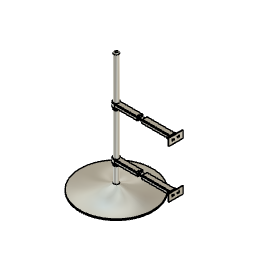
Base & Stand & Arms (Current) v10 (Autodesk Fusion 360 design; units mm, degrees)
Autodesk Fusion 360 part; units mm, degrees
sketch "Sketch1" plane through (0, 0, 0) normal (0, 1, 0) x (1, 0, 0) in component "Base"
  line L0 (0, 0) -> (0, -5)
  line L1 (0, -5) -> (5, -5)
  line L2 (5, -5) -> (5, -15)
  line L3 (5, -15) -> (10, -15)
  line L4 (10, -15) -> (10, -30)
  line L5 (0, 0) -> (150, 0)
  line L6 (150, 0) -> (150, -5)
  arc A0 (150, -5) -> (10, -30) centre (184.7311, -603.994) ccw
  dimension "d1" = 150
  dimension "d2" = 5
  dimension "d3" = 5
  dimension "d4" = 10
  dimension "d5" = 10
  dimension "d6" = 30
  dimension "d7" = 600
  dimension "d8" = 5
  constraint coincident L0.start L5.start
  constraint vertical L0
  constraint perpendicular L0 L1
  constraint perpendicular L1 L2
  constraint perpendicular L2 L3
  constraint perpendicular L3 L4
  constraint perpendicular L0 L5
  constraint perpendicular L5 L6
  measures "d1" distance of L0.start L5.end
  measures "d2" distance of L0.start L0.end
  measures "d3" distance of L0.end L1.end
  measures "d4" distance of L1.end L2.end
  measures "d5" horizontal distance of L0.start L3.end
  measures "d6" vertical distance of L0.start L4.end
  measures "d7" radius of A0
  measures "d8" distance of L5.end L6.end
revolve "Revolve1" add sketch "Sketch1" angle 360 about axis through (0, 0, 1.75) along (0, 0, 1) makes body 1 in component "Base"
thread "Thread1" "ISO Metric profile 10.0 M10x1.5 6H" major diameter 10.198 minor diameter 8.526 pitch 1.5 angle 60 resizes the face on face at (4.9938, -0.2492, 8.3333) on bodies 1 in component "Base"
sketch "Sketch1 (2)" plane through (0, 0, 0) normal (0, 1, 0) x (1, 0, 0) in component "Stand"
  line L0 (-150, -5) -> (150, -5)
  line L1 (-10, -30) -> (10, -30)
  line L2 (-10, -30) -> (10, -30)
  line L3 (-10, -15) -> (10, -15)
  line L4 (-10, -15) -> (10, -15)
  line L5 (-4.263, -15) -> (4.263, -15)
  line L6 (-4.263, -15) -> (4.263, -15)
  line L7 (-4.263, -5) -> (4.263, -5)
  line L8 (-4.263, -5) -> (4.263, -5)
  line L9 (-150, 0) -> (150, 0)
  line L10 (-150, -5) -> (150, -5)
  line L11 (0, -5) -> (4.263, -5)
  line L12 (4.263, -15) -> (10, -15)
  line L13 (10, -30) -> (10, -15)
  line L14 (4.263, -15) -> (4.263, -5)
  line L15 (10, -30) -> (10, -500)
  line L16 (10, -500) -> (0, -500)
  line L17 (0, -500) -> (0, -5)
  point P0 (0, -5)
  dimension "d10" = 500
  constraint midpoint L10 P0
  constraint coincident P0 L11.start
  constraint coincident L7.end L8.end
  constraint coincident L5.end L6.end
  constraint coincident L3.end L4.end
  constraint coincident L1.end L2.end
  constraint perpendicular L1 L15
  constraint perpendicular L15 L16
  constraint perpendicular L7 L17
  measures "d10" distance of L9 L15.end
revolve "Revolve1'" add sketch "Sketch1 (2)" angle 360 about axis through (0, 0, 500) along (0, 0, -1) separate body makes body 2 in component "Stand"
thread "Thread1'" "ISO Metric profile 9.0 M9x1 6g" major diameter 8.884 minor diameter 7.744 pitch 1 angle 60 resizes the face on face at (4.2577, 0.2125, 11.6667) on bodies 2 in component "Stand"
sketch "Sketch1 (3)" plane through (0, 0, 0) normal (0, 1, 0) x (1, 0, 0) in component "Connection part1 & Arm1"
  line L0 (-10, -15) -> (10, -15)
  line L1 (-10, -500) -> (10, -500)
  line L2 (-150, -5) -> (150, -5)
  line L3 (-10, -30) -> (10, -30)
  line L4 (-150, -5) -> (150, -5)
  line L5 (-150, 0) -> (150, 0)
  line L6 (-150, -5) -> (150, -5)
  line L7 (10, -100) -> (11, -100)
  line L8 (11, -100) -> (11, -105)
  line L9 (11, -105) -> (13, -105)
  line L10 (13, -105) -> (13, -120)
  line L11 (13, -120) -> (10, -120)
  line L12 (10, -120) -> (10, -100)
  line L13 (0, -1.75) -> (0, -22.5)
  point P0 (10, -100)
  dimension "d12" = 100
  dimension "d13" = 1
  dimension "d14" = 5
  dimension "d15" = 2
  dimension "d16" = 15
  dimension "d17" = 10
  dimension "d18" = 20
  constraint coincident P0 L7.start
  constraint horizontal L7
  constraint perpendicular L7 L8
  constraint perpendicular L8 L9
  constraint perpendicular L9 L10
  constraint perpendicular L10 L11
  measures "d12" distance of L5 P0
  measures "d13" distance of P0 L7.end
  measures "d14" distance of L7.end L8.end
  measures "d15" distance of L8.end L9.end
  measures "d16" distance of L9.end L10.end
  measures "d17" distance of P0 L13
  measures "d18" distance of L11.end P0
revolve "Revolve1''" add sketch "Sketch1 (3)" angle 360 about axis through (0, 0, 1.75) along (0, 0, 1) separate body makes body 3 in component "Connection part1 & Arm1"
thread "Thread1''" "ISO Metric profile 22.0 M22x1 6g" major diameter 21.884 minor diameter 20.741 pitch 1 angle 60 resizes the face on face at (10.9863, -0.5483, 101.6667) on bodies 3 in component "Connection part1 & Arm1"
sketch "Sketch1 (4)" plane through (0, 0, 0) normal (0, 1, 0) x (1, 0, 0) in component "Connection part2"
  line L0 (-13, -105) -> (13, -105)
  line L1 (-13, -120) -> (13, -120)
  line L2 (-10.942, -100) -> (10.942, -100)
  line L3 (-10.942, -105) -> (10.942, -105)
  line L4 (-150, -5) -> (150, -5)
  line L5 (-10, -30) -> (10, -30)
  line L6 (-150, 0) -> (150, 0)
  line L7 (-150, -5) -> (150, -5)
  line L8 (10.942, -100) -> (10.942, -105)
  line L9 (13, -105) -> (10.942, -105)
  line L10 (10.942, -100) -> (10, -100)
  line L11 (10, -100) -> (10, -95)
  arc A0 (10, -95) -> (13, -105) centre (59.1296, -85.7111) ccw
  point P0 (10.942, -100)
  dimension "d20" = 5
  dimension "d21" = 0.942
  dimension "d22" = 50
  constraint coincident P0 L2.end
  constraint coincident L3.end L8.end
  constraint coincident L0.end L9.start
  constraint coincident L2 L10.end
  constraint perpendicular L8 L10
  constraint perpendicular L10 L11
  measures "d20" distance of L10.end L11.end
  measures "d21" distance of P0 L10.end
  measures "d22" radius of A0
revolve "Revolve1'''" add sketch "Sketch1 (4)" angle 360 about axis through (0, 0, 1.75) along (0, 0, 1) separate body makes body 4 in component "Connection part2"
thread "Thread1'''" "ISO Metric profile 24.0 M24x1.5 6H" major diameter 24.2083 minor diameter 22.5262 pitch 1.5 angle 60 resizes the face on face at (10.9284, -0.5454, 101.6667) on bodies 4 in component "Connection part2"
sketch "Sketch2" plane through (0, 0, 0) normal (0, 1, 0) x (1, 0, 0) in component "Connection part1 & Arm1"
  line L0 (-13, -105) -> (13, -105)
  line L1 (-13, -120) -> (13, -120)
  line L2 (-13, -105) -> (13, -105)
  line L3 (11.2631, -100.161) -> (-11.2631, -100.161)
  line L4 (-11.2148, -100) -> (11.2148, -100)
  line L5 (-10, -95) -> (10, -95)
  line L6 (-10, -15) -> (10, -15)
  line L7 (-10, -500) -> (10, -500)
  line L8 (-150, -5) -> (150, -5)
  line L9 (-10, -30) -> (10, -30)
  line L10 (-150, -5) -> (150, -5)
  line L11 (-150, 0) -> (150, 0)
  line L12 (-150, -5) -> (150, -5)
  line L13 (0, -105) -> (0, -120)
  line L14 (0, -120) -> (100, -120)
  line L15 (0, -105) -> (100, -105)
  line L16 (100, -105) -> (100, -120)
  point P0 (0, -105)
  dimension "d24" = 100
  dimension "d25" = 15
  constraint midpoint L0 P0
  constraint coincident P0 L13.start
  constraint perpendicular L2 L13
  constraint perpendicular L13 L14
  constraint perpendicular L13 L15
  constraint perpendicular L14 L16
  measures "d24" distance of L13.end L14.end
  measures "d25" distance of L14.end L15.end
extrude "Extrude1" add sketch "Sketch2" along normal mid plane 24 bodies 3 in component "Connection part1 & Arm1"
sketch "Sketch3" plane through (0, 0, 120) normal (0, 0, 1) x (-1, 0, 0) in component "Connection part1 & Arm1"
  arc A0 (0, -10) -> (0, 10) centre (0, 0) ccw
  line L0 (0, -10) -> (0, 10)
  line L1 (-5, 12) -> (-100, 12)
  line L2 (-100, 12) -> (-100, -12)
  line L3 (-100, -12) -> (-5, -12)
  arc A1 (-5, -12) -> (-5, 12) centre (0, 0) ccw
  arc A2 (0, 10) -> (0, -10) centre (0, 0) ccw
  line L4 (0, -10) -> (0, 10)
  constraint coincident A0.centre A1.centre
  constraint coincident A0.start L0.start
  constraint parallel L0 L4
extrude "Extrude2" cut sketch "Sketch3" against normal blind 15 contours L0 A2 L4 bodies 3 in component "Connection part1 & Arm1"
sketch "Sketch4" plane through (100, 0, 0) normal (1, 0, 0) x (0, 1, 0) in component "Connection part1 & Arm1"
  line L0 (-12, 105) -> (12, 105)
  line L1 (12, 105) -> (12, 120)
  line L2 (12, 120) -> (-12, 120)
  line L3 (-12, 120) -> (-12, 105)
  circle A0 centre (0, 112.5) radius 6
  point P0 (0, 112.5)
  dimension "d30" = 7.5
  dimension "d31" = 12
  dimension "d32" = 12
  constraint coincident P0 A0.centre
  measures "d30" distance of L2 P0
  measures "d31" distance of L1 P0
  measures "d32" diameter of A0
extrude "Extrude3" cut sketch "Sketch4" against normal blind 8 contours A0 bodies 3 in component "Connection part1 & Arm1"
sketch "Sketch5" plane through (92, 0, 0) normal (1, 0, 0) x (0, 1, 0) in component "Connection part1 & Arm1"
  circle A0 centre (0, 112.5) radius 6
  circle A1 centre (0, 112.5) radius 2.5
  dimension "d35" = 5
  constraint concentric A0 A1
  measures "d35" diameter of A1
extrude "Extrude4" cut sketch "Sketch5" against normal blind 5 contours A1 bodies 3 in component "Connection part1 & Arm1"
thread "Thread2" "ISO Metric profile 6.0 M6x1 6H" major diameter 6.147 minor diameter 5.035 pitch 1 angle 60 resizes the face on face at (88.6667, 2.3492, 111.645) on bodies 3 in component "Connection part1 & Arm1"
sketch "Sketch1 (5)" plane through (0, 0, 0) normal (0, 1, 0) x (1, 0, 0) in component "Connection part3"
  line L0 (5, -120) -> (5, -105)
  line L1 (5, -105) -> (100, -105)
  line L2 (100, -105) -> (100, -120)
  line L3 (100, -120) -> (5, -120)
  line L4 (5, -120) -> (100, -120)
  line L5 (100, -120) -> (5, -120)
  line L6 (-13, -120) -> (5, -120)
  line L7 (-10, -120) -> (10, -120)
  line L8 (92, -106.5) -> (92, -118.5)
  line L9 (100, -106.5) -> (100, -118.5)
  line L10 (100, -106.5) -> (100, -118.5)
  line L11 (100, -105) -> (100, -120)
  line L12 (100, -120) -> (100, -105)
  line L13 (92, -109.9825) -> (92, -115.0175)
  line L14 (92, -106.5) -> (92, -118.5)
  line L15 (87, -109.9825) -> (87, -115.0175)
  line L16 (92, -109.9825) -> (92, -115.0175)
  line L17 (87, -109.9825) -> (87, -115.0175)
  line L18 (87, -112.5) -> (105, -112.5)
  line L19 (87, -112.5) -> (87, -109.9825)
  line L20 (92, -109.9825) -> (92, -106.5)
  line L21 (92, -109.9825) -> (87, -109.9825)
  line L22 (87, -112.5) -> (87, -109.9825)
  line L23 (92, -109.9825) -> (92, -106.5)
  line L24 (92, -106.5) -> (100, -106.5)
  line L25 (100, -106.5) -> (105, -106.5)
  line L26 (105, -112.5) -> (105, -106.5)
  point P0 (87, -112.5)
  dimension "d38" = 5
  dimension "d39" = 18
  constraint midpoint L15 P0
  constraint coincident P0 L18.start
  constraint perpendicular L12 L18
  constraint coincident L15.start L17.start
  constraint coincident L13.start L16.start
  constraint coincident L8.start L14.start
  constraint coincident L9.start L10.start
  constraint perpendicular L11 L25
  measures "d38" distance of L9.start L25.end
  measures "d39" distance of P0 L18.end
revolve "Revolve1''''" add sketch "Sketch1 (5)" angle 360 about axis through (87, 0, 112.5) along (1, 0, 0) separate body contours L2 L9 L10 L11 L12 L18 L25 L26 | L2 L8 L9 L10 L11 L12 L13 L14 L16 L18 L20 L23 L24 | L8 L13 L14 L15 L16 L17 L18 L19 L21 L22 makes body 5 in component "Connection part3"
sketch "Sketch2 (2)" plane through (0, 0, 0) normal (0, 1, 0) x (1, 0, 0) in component "Connection part3"
  line L0 (92, -118.5) -> (92, -106.5)
  line L1 (105, -118.5) -> (105, -106.5)
  arc A0 (105, -118.5) -> (111, -112.5) centre (105, -112.5) ccw
  line L2 (111, -112.5) -> (105, -112.5)
  line L3 (105, -118.5) -> (105, -112.5)
  point P0 (105, -112.5)
  constraint midpoint L1 P0
  constraint coincident L1.start A0.start
  constraint coincident P0 A0.centre
  constraint perpendicular L1 L2
revolve "Revolve2" add sketch "Sketch2 (2)" angle 360 about axis through (87, 0, 112.5) along (1, 0, 0) bodies 5 in component "Connection part3"
sketch "Sketch3 (2)" plane through (0, 0, 0) normal (0, 1, 0) x (1, 0, 0) in component "Connection part3"
  line L0 (87, -115.0175) -> (87, -109.9825)
  line L1 (92, -118.5) -> (92, -115.0175)
  line L2 (92, -109.9825) -> (92, -106.5)
  arc A0 (105, -118.5) -> (105, -106.5) centre (105, -112.5) ccw
  line L3 (87, -115.0175) -> (92, -115.0175)
  line L4 (87, -109.9825) -> (92, -109.9825)
  line L5 (92, -118.5) -> (105, -118.5)
  line L6 (92, -106.5) -> (105, -106.5)
  circle A1 centre (108.5, -112.5) radius 1.5
  point P0 (105, -112.5)
  point P1 (108.5, -112.5)
  dimension "d42" = 3.5
  dimension "d43" = 3
  constraint coincident P0 A0.centre
  constraint coincident P1 A1.centre
  constraint horizontal P0 P1
  measures "d42" distance of P0 P1
  measures "d43" diameter of A1
extrude "Extrude1'" cut sketch "Sketch3 (2)" along normal through all and the other way through all contours A1 bodies 5 in component "Connection part3"
thread "Thread1''''" "ISO Metric profile 5.0 M5x0.8 6g" major diameter 4.901 minor diameter 3.9895 pitch 0.8 angle 60 resizes the face on face at (90.3333, 2.1148, 111.1341) on bodies 5 in component "Connection part3"
sketch "Sketch1 (6)" plane through (0, 0, 0) normal (0, 1, 0) x (1, 0, 0) in component "Arm2"
  spline S0 degree 3 poles (110, -112.5) (110, -112.3105) (109.9621, -112.1167) (109.8242, -111.7712) (109.7245, -111.619) (109.4765, -111.3419) (109.2992, -111.213) (108.9108, -111.0418) (108.6997, -111) (108.3147, -111) (108.1111, -111.0363) (107.7265, -111.198) (107.5455, -111.3235) (107.2851, -111.6039) (107.1795, -111.7631) (107.0368, -112.1182) (107, -112.3141) (107, -112.6859) (107.0368, -112.8818) (107.1795, -113.2369) (107.2851, -113.3961) (107.5455, -113.6765) (107.7265, -113.802) (108.1111, -113.9637) (108.3147, -114) (108.6997, -114) (108.9108, -113.9582) (109.2992, -113.787) (109.4765, -113.6581) (109.7245, -113.381) (109.8242, -113.2288) (109.9621, -112.8833) (110, -112.6895) (110, -112.5) knots 0 0 0 0 0.056857 0.056857 0.113714 0.113714 0.188792 0.188792 0.26387 0.26387 0.333535 0.333535 0.403199 0.403199 0.458977 0.458977 0.514754 0.514754 0.570532 0.570532 0.626309 0.626309 0.695974 0.695974 0.765638 0.765638 0.840717 0.840717 0.915795 0.915795 0.972652 0.972652 1.029508 1.029508 1.029508 1.029508
  line L0 (87, -114.9505) -> (87, -110.0495)
  line L1 (92, -118.5) -> (92, -114.9505)
  line L2 (92, -110.0495) -> (92, -106.5)
  arc A0 (105, -118.5) -> (105, -106.5) centre (105, -112.5) ccw
  line L3 (87, -114.9505) -> (92, -114.9505)
  line L4 (87, -110.0495) -> (92, -110.0495)
  line L5 (92, -118.5) -> (105, -118.5)
  line L6 (92, -106.5) -> (105, -106.5)
  circle A1 centre (108.5, -112.5) radius 1.5
  dimension "d45" = 3.5
  dimension "d46" = 3
  constraint horizontal A0.centre A1.centre
  measures "d45" distance of A0.centre A1.centre
  measures "d46" diameter of A1
extrude "Extrude1''" add sketch "Sketch1 (6)" along normal mid plane 16 separate body contours S0 A1 makes body 6 in component "Arm2"
sketch "Sketch2 (3)" plane through (0, -8, 0) normal (0, -1, 0) x (1, 0, 0) in component "Arm2"
  spline S0 degree 3 poles (110, 112.5) (110, 112.6895) (109.9621, 112.8833) (109.8242, 113.2288) (109.7245, 113.381) (109.4765, 113.6581) (109.2992, 113.787) (108.9108, 113.9582) (108.6997, 114) (108.3147, 114) (108.1111, 113.9637) (107.7265, 113.802) (107.5455, 113.6765) (107.2851, 113.3961) (107.1795, 113.2369) (107.0368, 112.8818) (107, 112.6859) (107, 112.3141) (107.0368, 112.1182) (107.1795, 111.7631) (107.2851, 111.6039) (107.5455, 111.3235) (107.7265, 111.198) (108.1111, 111.0363) (108.3147, 111) (108.6997, 111) (108.9108, 111.0418) (109.2992, 111.213) (109.4765, 111.3419) (109.7245, 111.619) (109.8242, 111.7712) (109.9621, 112.1167) (110, 112.3105) (110, 112.5) knots -1.029508 -1.029508 -1.029508 -1.029508 -0.972652 -0.972652 -0.915795 -0.915795 -0.840717 -0.840717 -0.765638 -0.765638 -0.695974 -0.695974 -0.626309 -0.626309 -0.570532 -0.570532 -0.514754 -0.514754 -0.458977 -0.458977 -0.403199 -0.403199 -0.333535 -0.333535 -0.26387 -0.26387 -0.188792 -0.188792 -0.113714 -0.113714 -0.056857 -0.056857 0 0 0 0
  spline S1 degree 3 poles (110, 112.5) (110, 112.6895) (109.9621, 112.8833) (109.8242, 113.2288) (109.7245, 113.381) (109.4765, 113.6581) (109.2992, 113.787) (108.9108, 113.9582) (108.6997, 114) (108.3147, 114) (108.1111, 113.9637) (107.7265, 113.802) (107.5455, 113.6765) (107.2851, 113.3961) (107.1795, 113.2369) (107.0368, 112.8818) (107, 112.6859) (107, 112.3141) (107.0368, 112.1182) (107.1795, 111.7631) (107.2851, 111.6039) (107.5455, 111.3235) (107.7265, 111.198) (108.1111, 111.0363) (108.3147, 111) (108.6997, 111) (108.9108, 111.0418) (109.2992, 111.213) (109.4765, 111.3419) (109.7245, 111.619) (109.8242, 111.7712) (109.9621, 112.1167) (110, 112.3105) (110, 112.5) knots 0 0 0 0 0.056857 0.056857 0.113714 0.113714 0.188792 0.188792 0.26387 0.26387 0.333535 0.333535 0.403199 0.403199 0.458977 0.458977 0.514754 0.514754 0.570532 0.570532 0.626309 0.626309 0.695974 0.695974 0.765638 0.765638 0.840717 0.840717 0.915795 0.915795 0.972652 0.972652 1.029508 1.029508 1.029508 1.029508
  line L0 (87, 110.0495) -> (87, 114.9505)
  line L1 (92, 106.5) -> (92, 110.0495)
  line L2 (92, 114.9505) -> (92, 118.5)
  arc A0 (105, 106.5) -> (105, 118.5) centre (105, 112.5) ccw
  line L3 (87, 110.0495) -> (92, 110.0495)
  line L4 (87, 114.9505) -> (92, 114.9505)
  line L5 (92, 106.5) -> (105, 106.5)
  line L6 (92, 118.5) -> (105, 118.5)
  spline S2 degree 3 poles (110, 112.5) (110, 112.3105) (109.9621, 112.1167) (109.8242, 111.7712) (109.7245, 111.619) (109.4765, 111.3419) (109.2992, 111.213) (108.9108, 111.0418) (108.6997, 111) (108.3147, 111) (108.1111, 111.0363) (107.7265, 111.198) (107.5455, 111.3235) (107.2851, 111.6039) (107.1795, 111.7631) (107.0368, 112.1182) (107, 112.3141) (107, 112.6859) (107.0368, 112.8818) (107.1795, 113.2369) (107.2851, 113.3961) (107.5455, 113.6765) (107.7265, 113.802) (108.1111, 113.9637) (108.3147, 114) (108.6997, 114) (108.9108, 113.9582) (109.2992, 113.787) (109.4765, 113.6581) (109.7245, 113.381) (109.8242, 113.2288) (109.9621, 112.8833) (110, 112.6895) (110, 112.5) knots 0 0 0 0 0.056857 0.056857 0.113714 0.113714 0.188792 0.188792 0.26387 0.26387 0.333535 0.333535 0.403199 0.403199 0.458977 0.458977 0.514754 0.514754 0.570532 0.570532 0.626309 0.626309 0.695974 0.695974 0.765638 0.765638 0.840717 0.840717 0.915795 0.915795 0.972652 0.972652 1.029508 1.029508 1.029508 1.029508
  line L7 (108.5, 112.5) -> (108.5, 111)
  line L8 (108.5, 112.5) -> (108.5, 114)
  line L9 (108.5, 114) -> (115.5, 114)
  line L10 (108.5, 111) -> (115.5, 111)
  line L11 (115.5, 111) -> (115.5, 114)
  point P0 (108.5, 112.5)
  dimension "d49" = 3.5
  dimension "d50" = 7
  dimension "d51" = 7
  constraint horizontal A0.centre P0
  constraint coincident P0 L7.start
  constraint coincident S2 L7.end
  constraint coincident S1 L7.end
  constraint coincident S0 L7.end
  constraint coincident S1 L8.end
  constraint coincident S2 L8.end
  constraint coincident S0 L8.end
  constraint parallel L2 L8
  constraint parallel L7 L8
  constraint perpendicular L8 L9
  constraint perpendicular L7 L10
  measures "d49" distance of A0.centre P0
  measures "d50" distance of L8.end L9.end
  measures "d51" distance of L7.end L10.end
extrude "Extrude2'" add sketch "Sketch2 (3)" against normal blind 2 separate body contours S0 S1 A0 S2 L9 L10 | A0 L9 L10 L11 makes body 7 in component "Arm2"
mirror "Mirror1" about plane through (0, 0, 0) normal (0, 1, 0) of bodies 7 makes body 8 in component "Arm2"
sketch "Sketch3 (3)" plane through (0, 0, 0) normal (0, 1, 0) x (1, 0, 0) in component "Arm2"
  line L0 (115.5, -111) -> (115.5, -114)
  line L1 (108.5, -114) -> (115.5, -114)
  spline S0 degree 3 poles (108.5, -114) (108.6997, -114) (108.9108, -113.9582) (109.2992, -113.787) (109.4765, -113.6581) (109.7245, -113.381) (109.8242, -113.2288) (109.9621, -112.8833) (110, -112.6895) (110, -112.5) (110, -112.3105) (109.9621, -112.1167) (109.8242, -111.7712) (109.7245, -111.619) (109.4765, -111.3419) (109.2992, -111.213) (108.9108, -111.0418) (108.6997, -111) (108.5, -111) knots -0.26387 -0.26387 -0.26387 -0.26387 -0.188792 -0.188792 -0.113714 -0.113714 -0.056857 -0.056857 0 0 0 0.056857 0.056857 0.113714 0.113714 0.188792 0.188792 0.26387 0.26387 0.26387 0.26387
  line L2 (108.5, -111) -> (115.5, -111)
  spline S1 degree 3 poles (110, -112.5) (110, -112.6895) (109.9621, -112.8833) (109.8242, -113.2288) (109.7245, -113.381) (109.4765, -113.6581) (109.2992, -113.787) (108.9108, -113.9582) (108.6997, -114) (108.3147, -114) (108.1111, -113.9637) (107.7265, -113.802) (107.5455, -113.6765) (107.2851, -113.3961) (107.1795, -113.2369) (107.0368, -112.8818) (107, -112.6859) (107, -112.3141) (107.0368, -112.1182) (107.1795, -111.7631) (107.2851, -111.6039) (107.5455, -111.3235) (107.7265, -111.198) (108.1111, -111.0363) (108.3147, -111) (108.6997, -111) (108.9108, -111.0418) (109.2992, -111.213) (109.4765, -111.3419) (109.7245, -111.619) (109.8242, -111.7712) (109.9621, -112.1167) (110, -112.3105) (110, -112.5) knots -1.029508 -1.029508 -1.029508 -1.029508 -0.972652 -0.972652 -0.915795 -0.915795 -0.840717 -0.840717 -0.765638 -0.765638 -0.695974 -0.695974 -0.626309 -0.626309 -0.570532 -0.570532 -0.514754 -0.514754 -0.458977 -0.458977 -0.403199 -0.403199 -0.333535 -0.333535 -0.26387 -0.26387 -0.188792 -0.188792 -0.113714 -0.113714 -0.056857 -0.056857 0 0 0 0
  line L3 (115.5, -112.5) -> (115.5, -120)
  line L4 (115.5, -112.5) -> (115.5, -105)
  line L5 (115.5, -120) -> (235.5, -120)
  line L6 (115.5, -105) -> (235.5, -105)
  line L7 (235.5, -105) -> (235.5, -120)
  point P0 (115.5, -112.5)
  dimension "d56" = 7.5
  dimension "d57" = 7.5
  dimension "d58" = 120
  dimension "d59" = 120
  constraint midpoint L0 P0
  constraint coincident P0 L3.start
  constraint perpendicular L1 L3
  constraint perpendicular L1 L4
  constraint perpendicular L3 L5
  constraint perpendicular L4 L6
  measures "d56" distance of P0 L3.end
  measures "d57" distance of P0 L4.end
  measures "d58" distance of L3.end L5.end
  measures "d59" distance of L4.end L6.end
extrude "Extrude3'" add sketch "Sketch3 (3)" along normal mid plane 24 contours L0 L3 L4 L5 L6 L7 bodies 7 8 in component "Arm2"
sketch "Sketch4 (2)" plane through (0, -12, 0) normal (0, -1, 0) x (1, 0, 0) in component "Arm2"
  line L0 (115.5, 120) -> (115.5, 105)
  line L1 (115.5, 105) -> (235.5, 105)
  line L2 (235.5, 105) -> (235.5, 120)
  line L3 (235.5, 120) -> (115.5, 120)
  circle A0 centre (229.5, 112.5) radius 4
  point P0 (229.5, 112.5)
  dimension "d62" = 6
  dimension "d63" = 8
  dimension "d64" = 7.5
  constraint coincident P0 A0.centre
  measures "d62" distance of L2 P0
  measures "d63" diameter of A0
  measures "d64" distance of L3 P0
extrude "Extrude4'" cut sketch "Sketch4 (2)" along normal through all and the other way through all contours A0 bodies 7 in component "Arm2"
sketch "Sketch1 (7)" plane through (0, 0, 0) normal (0, 1, 0) x (1, 0, 0) in component "Connection part 4"
  circle A0 centre (229.5, -112.5) radius 4
  line L0 (115.5, -120) -> (115.5, -114)
  line L1 (115.5, -111) -> (115.5, -105)
  line L2 (115.5, -105) -> (235.5, -105)
  line L3 (235.5, -105) -> (235.5, -120)
  line L4 (235.5, -120) -> (115.5, -120)
  line L5 (108.5, -114) -> (115.5, -114)
  spline S0 degree 3 poles (108.5, -114) (108.6997, -114) (108.9108, -113.9582) (109.2992, -113.787) (109.4765, -113.6581) (109.7245, -113.381) (109.8242, -113.2288) (109.9621, -112.8833) (110, -112.6895) (110, -112.5) (110, -112.3105) (109.9621, -112.1167) (109.8242, -111.7712) (109.7245, -111.619) (109.4765, -111.3419) (109.2992, -111.213) (108.9108, -111.0418) (108.6997, -111) (108.5, -111) knots -0.26387 -0.26387 -0.26387 -0.26387 -0.188792 -0.188792 -0.113714 -0.113714 -0.056857 -0.056857 0 0 0 0.056857 0.056857 0.113714 0.113714 0.188792 0.188792 0.26387 0.26387 0.26387 0.26387
  line L6 (108.5, -111) -> (115.5, -111)
  circle A1 centre (229.5, -112.5) radius 4
  dimension "d66" = 8
  constraint concentric A0 A1
  measures "d66" diameter of A1
extrude "Extrude1'''" add sketch "Sketch1 (7)" along normal mid plane 32 separate body contours A0 A1 makes body 9 in component "Connection part 4"
sketch "Sketch2 (4)" plane through (0, -16, 0) normal (0, -1, 0) x (1, 0, 0) in component "Connection part 4"
  circle A0 centre (229.5, 112.5) radius 4
  circle A1 centre (229.5, 112.5) radius 4
  line L0 (229.5, 112.5) -> (229.5, 116.5)
  line L1 (229.5, 112.5) -> (229.5, 108.5)
  line L2 (229.5, 116.5) -> (245.5, 116.5)
  line L3 (229.5, 108.5) -> (245.5, 108.5)
  line L4 (245.5, 116.5) -> (245.5, 108.5)
  dimension "d69" = 16
  dimension "d70" = 16
  constraint coincident A0.centre A1.centre
  constraint coincident A1 L0.end
  constraint vertical L0
  constraint coincident A1 L1.end
  constraint parallel L0 L1
  constraint perpendicular L0 L2
  constraint perpendicular L1 L3
  measures "d69" distance of L0.end L2.end
  measures "d70" distance of L1.end L3.end
extrude "Extrude2''" add sketch "Sketch2 (4)" against normal blind 4 separate body contours A0 A1 L2 L3 L4 makes body 10 in component "Connection part 4"
mirror "Mirror1'" about plane through (0, 0, 0) normal (0, 1, 0) of bodies 10 makes body 11 in component "Connection part 4"
sketch "Sketch3 (4)" plane through (0, 0, 0) normal (0, 1, 0) x (1, 0, 0) in component "Connection part 4"
  line L0 (245.5, -116.5) -> (245.5, -108.5)
  line L1 (229.5, -116.5) -> (245.5, -116.5)
  arc A0 (229.5, -116.5) -> (229.5, -108.5) centre (229.5, -112.5) ccw
  line L2 (229.5, -108.5) -> (245.5, -108.5)
  line L3 (245.5, -112.5) -> (245.5, -127.5)
  line L4 (245.5, -112.5) -> (245.5, -97.5)
  line L5 (245.5, -127.5) -> (247, -127.5)
  line L6 (245.5, -97.5) -> (247, -97.5)
  line L7 (247, -97.5) -> (247, -127.5)
  point P0 (245.5, -112.5)
  dimension "d75" = 15
  dimension "d76" = 15
  dimension "d77" = 1.5
  constraint midpoint L0 P0
  constraint coincident P0 L3.start
  constraint parallel L0 L3
  constraint perpendicular L2 L4
  constraint perpendicular L3 L5
  constraint perpendicular L4 L6
  constraint perpendicular L5 L7
  measures "d75" distance of P0 L3.end
  measures "d76" distance of P0 L4.end
  measures "d77" distance of L3.end L5.end
extrude "Extrude3''" add sketch "Sketch3 (4)" along normal mid plane 60 contours L0 L3 L4 L5 L6 L7 bodies 10 11 in component "Connection part 4"
sketch "Sketch4 (3)" plane through (247, 0, 0) normal (1, 0, 0) x (0, 1, 0) in component "Connection part 4"
  line L0 (-30, 97.5) -> (30, 97.5)
  line L1 (30, 97.5) -> (30, 127.5)
  line L2 (30, 127.5) -> (-30, 127.5)
  line L3 (-30, 127.5) -> (-30, 97.5)
  circle A0 centre (-7.5, 112.5) radius 2.5
  circle A1 centre (7.5, 112.5) radius 2.5
  point P0 (-7.5, 112.5)
  point P1 (7.5, 112.5)
  dimension "d80" = 15
  dimension "d81" = 22.5
  dimension "d82" = 15
  dimension "d83" = 5
  dimension "d84" = 5
  constraint horizontal P0 P1
  constraint coincident P0 A0.centre
  constraint coincident P1 A1.centre
  measures "d80" distance of P0 P1
  measures "d81" distance of L3 P0
  measures "d82" distance of L2 P0
  measures "d83" diameter of A0
  measures "d84" diameter of A1
extrude "Extrude4''" cut sketch "Sketch4 (3)" against normal blind 1.5 contours A0 | A1 bodies 10 in component "Connection part 4"
ref_plane "WorkPlane1" through (0, 0, 110) normal (0, 0, 1) x (1, 0, 0)
sketch "Sketch1 (8)" plane through (0, 0, 110) normal (0, 0, 1) x (1, 0, 0)
  circle A0 centre (0, 0) radius 10
  dimension "d92" = 20
  constraint coincident A0.centre origin
  measures "d92" diameter of A0
ref_plane "WorkPlane2" through (0, 0, 310) normal (0, 0, 1) x (1, 0, 0)
sketch "Sketch2 (5)" plane through (0, 0, 310) normal (0, 0, 1) x (1, 0, 0)
  circle A0 centre (0, 0) radius 10
  dimension "d98" = 20
  constraint coincident A0.centre origin
  measures "d98" diameter of A0
fillet "Fillet1" radius 5 1 edges at (-9.3233, -3.6162, 500) on bodies 2 in component "Stand"
thread "Thread1'''''" "ISO Metric profile 6.0 M6x1 6H" major diameter 6.147 minor diameter 5.035 pitch 1 angle 60 resizes the face on face at (246, -5.1508, 111.6449) on bodies 10 in component "Connection part 4"
thread "Thread2'" "ISO Metric profile 6.0 M6x1 6H" major diameter 6.147 minor diameter 5.035 pitch 1 angle 60 resizes the face on face at (246, 5.1508, 111.6449) on bodies 10 in component "Connection part 4"
thread "Thread3" "ISO Metric profile 6.0 M6x1 6H" major diameter 6.147 minor diameter 5.035 pitch 1 angle 60 resizes the face on face at (246, -9.8198, 113.4779) on bodies 10 in component "Connection part 4"
thread "Thread4" "ISO Metric profile 6.0 M6x1 6H" major diameter 6.147 minor diameter 5.035 pitch 1 angle 60 resizes the face on face at (246, 5.1802, 113.4779) on bodies 10 in component "Connection part 4"
fillet "Fillet1'" radius 2.5 8 edges at (175.5, 12, 120) (175.5, -12, 120) (175.5, -12, 105) (175.5, 12, 105) (175.5, -12, 120) (175.5, -12, 105) (175.5, 12, 120) (175.5, 12, 105) on bodies 7 in component "Arm2"
fillet "Fillet1''" radius 2.5 8 edges at (52.5, -12, 120) (52.5, -12, 105) (52.5, 12, 120) (52.5, 12, 105) (52.5, -12, 120) (52.5, -12, 105) (52.5, 12, 120) (52.5, 12, 105) on bodies 3 in component "Connection part1 & Arm1"
fillet "Fillet2" radius 2.5 32 edges at (235.5, 12, 112.5) (235.5, 11.2678, 105.7322) (235.5, 0, 105) (235.5, -11.2678, 105.7322) (235.5, -12, 112.5) (235.5, -11.2678, 119.2678) (235.5, 0, 120) (235.5, 11.2678, 119.2678) (115.5, 11.2678, 119.2678) (115.5, 12, 112.5) (115.5, 11.2678, 105.7322) (115.5, 0, 105) (115.5, -11.2678, 105.7322) (115.5, -12, 112.5) (115.5, -11.2678, 119.2678) (115.5, 0, 120) (235.5, 12, 112.5) (235.5, 11.2678, 105.7322) (235.5, 0, 105) (235.5, -11.2678, 105.7322) (235.5, -12, 112.5) (235.5, -11.2678, 119.2678) (235.5, 0, 120) (235.5, 11.2678, 119.2678) (115.5, -11.2678, 105.7322) (115.5, 0, 105) (115.5, 11.2678, 105.7322) (115.5, 12, 112.5) (115.5, 11.2678, 119.2678) (115.5, 0, 120) (115.5, -11.2678, 119.2678) (115.5, -12, 112.5) on bodies 7 in component "Arm2"
fillet "Fillet2'" radius 2.5 16 edges at (100, 12, 112.5) (100, 11.2678, 105.7322) (100, 0, 105) (100, -11.2678, 105.7322) (100, -12, 112.5) (100, -11.2678, 119.2678) (100, 0, 120) (100, 11.2678, 119.2678) (100, 12, 112.5) (100, 11.2678, 105.7322) (100, 0, 105) (100, -11.2678, 105.7322) (100, -12, 112.5) (100, -11.2678, 119.2678) (100, 0, 120) (100, 11.2678, 119.2678) on bodies 3 in component "Connection part1 & Arm1"
component "Base" placed x (1, 0, 0) y (0, 1, 0) z (0, 0, 1) at (0, 0, 0)
component "Stand" placed x (1, 0, 0) y (0, 1, 0) z (0, 0, 1) at (0, 0, 0)
component "Connection part1 & Arm1" placed x (1, 0, 0) y (0, 1, 0) z (0, 0, 1) at (0, 0, 0)
component "Connection part2" placed x (1, 0, 0) y (0, 1, 0) z (0, 0, 1) at (0, 0, -0.161)
component "Connection part3" placed x (1, 0, 0) y (0, 1, 0) z (0, 0, 1) at (0, 0, 0)
component "Arm2" placed x (1, 0, 0) y (0, 1, 0) z (0, 0, 1) at (0, 0, 0)
component "Connection part 4" placed x (1, 0, 0) y (0, 1, 0) z (0, 0, 1) at (0, 0, 0)
component "Connection part1 & Arm1" placed x (1, 0, 0) y (0, 1, 0) z (0, 0, 1) at (0, 0, 200)
component "Connection part2" placed x (1, 0, 0) y (0, 1, 0) z (0, 0, 1) at (0, 0, 199.839)
component "Connection part3" placed x (1, 0, 0) y (0, 1, 0) z (0, 0, 1) at (0, 0, 200)
component "Arm2" placed x (1, 0, 0) y (0, 1, 0) z (0, 0, 1) at (0, 0, 200)
component "Connection part 4" placed x (1, 0, 0) y (0, 1, 0) z (0, 0, 1) at (0, 0, 200)
